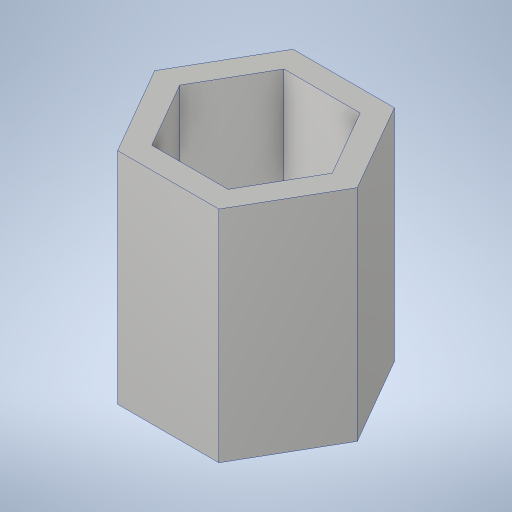
# Autodesk Inventor part: 3-8 1-2 adaptor
Saved by Autodesk Inventor 2023.4 (Build 274418000, 418)
## iProperties
Created: 2025-01-10
Part Number: 3-8 1-2 adaptor
Material: Aluminum 6061
Document SubType Name: Modeling
Designer: mavericks
Density: 2.7 g/cm^3
Appearance: Aluminum - Flat
Author: mavericks
Autodesk Inventor part; units mm, degrees
ref_plane "YZ Plane" through (0, 0, 0) normal (1, 0, 0) x (0, 1, 0)
ref_plane "XZ Plane" through (0, 0, 0) normal (0, 1, 0) x (-1, 0, 0)
ref_plane "XY Plane" through (0, 0, 0) normal (0, 0, 1) x (1, 0, 0)
sketch "Sketch1" plane through (0, 0, 0) normal (0, 1, 0) x (-1, 0, 0)
  line L0 (-5.5108, 0) -> (-2.7554, 4.7725)
  line L1 (-2.7554, 4.7725) -> (2.7554, 4.7725)
  line L2 (2.7554, 4.7725) -> (5.5108, 0)
  line L3 (5.5108, 0) -> (2.7554, -4.7725)
  line L4 (2.7554, -4.7725) -> (-2.7554, -4.7725)
  line L5 (-2.7554, -4.7725) -> (-5.5108, 0)
  line L6 (-3.6604, -6.34) -> (3.6604, -6.34)
  line L7 (3.6604, -6.34) -> (7.3208, 0)
  line L8 (7.3208, 0) -> (3.6604, 6.34)
  line L9 (3.6604, 6.34) -> (-3.6604, 6.34)
  line L10 (-3.6604, 6.34) -> (-7.3208, 0)
  line L11 (-7.3208, 0) -> (-3.6604, -6.34)
  point P0 (0, 0)
  point P1 (0, 0)
  dimension "d0" = 9.545
  dimension "d1" = 12.68
  constraints: 24 end point, 1 coincident, 1 horizontal, 18 other
  measures "d0" distance between parallel lines of L1 L4
  measures "d1" distance between parallel lines of L9 L6
extrude "Extrusion1" add sketch "Sketch1" along normal mid plane 15.875
body "Solid1"
